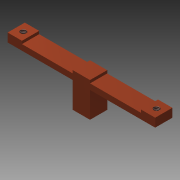
# Autodesk Inventor part: top_conductor
Saved by Autodesk Inventor 2014 SP1 (Build 180222100, 222)
## iProperties
Created: 2016-08-31
Part Number: top_conductor
Material: Copper, Alloy
Document SubType Name: Modeling
Designer: tguillod
Density: 7.58 g/cm^3
Appearance: Copper - Satin
Author: tguillod
Autodesk Inventor part; units mm, degrees
ref_plane "YZ Plane" through (0, 0, 0) normal (1, 0, 0) x (0, 1, 0)
ref_plane "XZ Plane" through (0, 0, 0) normal (0, 1, 0) x (-1, 0, 0)
ref_plane "XY Plane" through (0, 0, 0) normal (0, 0, 1) x (1, 0, 0)
sketch "Sketch1" plane through (0, 0, 0) normal (0, 0, 1) x (1, 0, 0)
  line L0 (0, 0) -> (51.5, 0)
  line L1 (51.5, 0) -> (51.5, 6)
  line L2 (51.5, 6) -> (0, 6)
  line L3 (0, 6) -> (0, 0)
  dimension "d0" = 6
  dimension "d1" = 51.5
  constraints: 8 end point, 2 parallel, 1 horizontal, 1 perpendicular
  measures "d0" distance of L0.end L1.end
  measures "d1" distance of L1.end L2.end
extrude "Extrusion1" add sketch "Sketch1" along normal blind 2
sketch "Sketch2" plane through (0, 0, 2) normal (0, 0, 1) x (1, 0, 0)
  line L0 (0, 0) -> (51.5, 0) projected
  line L1 (51.5, 0) -> (51.5, 6) projected
  line L2 (51.5, 6) -> (0, 6) projected
  line L3 (0, 6) -> (0, 0) projected
  line L4 (0, 6) -> (5, 6)
  line L5 (5, 6) -> (5, 0)
  line L6 (5, 0) -> (0, 0)
  line L7 (0, 0) -> (0, 6)
  line L8 (22.75, 6) -> (28.75, 6)
  line L9 (28.75, 6) -> (28.75, 0)
  line L10 (28.75, 0) -> (22.75, 0)
  line L11 (22.75, 0) -> (22.75, 6)
  line L12 (51.5, 6) -> (46.5, 6)
  line L13 (46.5, 6) -> (46.5, 0)
  line L14 (46.5, 0) -> (51.5, 0)
  line L15 (51.5, 0) -> (51.5, 6)
  dimension "d4" = 5
  dimension "d5" = 5
  dimension "d7" = 17.75
  dimension "d8" = 17.75
  dimension "d41" = 6
  constraints: 24 end point, 6 parallel, 4 point on line, 3 horizontal, 3 perpendicular
  measures "d4" distance between parallel lines of L3 L5
  measures "d5" distance between parallel lines of L1 L13
  measures "d7" distance between parallel lines of L11 L5
  measures "d8" distance between parallel lines of L13 L9
  measures "d41" distance between parallel lines of L9 L11
extrude "Extrusion2" add sketch "Sketch2" along normal blind 1 contours L3 L2 L5 L0 | L11 L2 L9 L0 | L13 L2 L1 L0
sketch "Sketch5" plane through (0, 0, 0) normal (0, 0, -1) x (-1, 0, 0)
  line L0 (0, 0) -> (-51.5, 0) projected
  line L1 (0, 6) -> (0, 0) projected
  line L2 (-51.5, 6) -> (0, 6) projected
  line L3 (-51.5, 0) -> (-51.5, 6) projected
  line L4 (-25.75, 6) -> (-25.75, 0) construction
  line L5 (-51.5, 3) -> (0, 3) construction
  line L6 (-28.75, 6) -> (-22.75, 6)
  line L7 (-22.75, 6) -> (-22.75, 0)
  line L8 (-22.75, 0) -> (-28.75, 0)
  line L9 (-28.75, 0) -> (-28.75, 6)
  line L10 (-28.75, 6) -> (-22.75, 0) construction
  line L11 (-22.75, 6) -> (-28.75, 0) construction
  point P0 (-25.75, 3)
  dimension "d19" = 6
  constraints: 16 end point, 7 midpoint, 2 parallel, 1 horizontal, 1 perpendicular, 1 point on line
  measures "d19" distance of L6.start L6.end
extrude "Extrusion3" add sketch "Sketch5" along normal blind 9 contours L0 L9 L2 L7
sketch "Sketch6" plane through (0, 0, -9) normal (0, 0, -1) x (-1, 0, 0)
  line L0 (-22.75, 0) -> (-22.75, 6) projected
  line L1 (-22.75, 6) -> (-28.75, 6) projected
  line L2 (-28.75, 6) -> (-28.75, 0) projected
  line L3 (-28.75, 0) -> (-22.75, 0) projected
  line L4 (-28.75, 3) -> (-22.75, 3) construction
  line L5 (-25.75, 6) -> (-25.75, 0) construction
  point P0 (0, 0)
  point P1 (-25.75, 3)
  constraints: 5 midpoint, 4 end point
hole "Hole2" at (25.75, 3, -9) direction (0, 0, 1) diameter 2.459 depth 8 tip angle 118 thread size "M3x0.5" class "6H" standard "ISO Metric profile"
sketch "Sketch7" plane through (0, 0, 0) normal (0, 0, -1) x (-1, 0, 0)
  line L0 (0, 6) -> (0, 0) projected
  line L1 (0, 0) -> (-22.75, 0) projected
  line L2 (0, 6) -> (0, 0) projected
  line L3 (-51.5, 0) -> (-51.5, 6) projected
  line L4 (-51.5, 6) -> (-28.75, 6) projected
  line L5 (-51.5, 3) -> (0, 3) construction
  line L6 (-22.75, 6) -> (-22.75, 0) projected
  line L7 (-28.75, 6) -> (-22.75, 6) projected
  line L8 (-28.75, 0) -> (-28.75, 6) projected
  line L9 (-28.75, 0) -> (-51.5, 0) projected
  line L10 (-22.75, 6) -> (0, 6) projected
  line L11 (-22.75, 0) -> (-28.75, 0) projected
  point P0 (-49, 3)
  point P1 (-2.5, 3)
  dimension "d31" = 2.5
  dimension "d32" = 2.5
  constraints: 2 end point, 2 midpoint, 2 point on line
  measures "d31" distance from line of L3 point (-49, 3)
  measures "d32" distance from line of L0 point (-2.5, 3)
hole "Hole3" at (49, 3, 0) at (2.5, 3, 0) direction (0, 0, 1) diameter 2.013 depth 3 tip angle 118 thread size "M2.5x0.45" class "6H" standard "ISO Metric profile"
body "Solid1"
